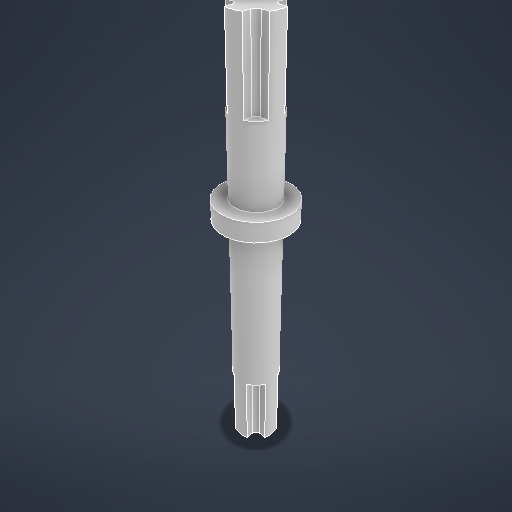
# Autodesk Inventor part: diff_gear_holder_2
Saved by Autodesk Inventor 2025 (Build 290162000, 162)
## iProperties
Created: 2024-07-25
Part Number: diff_gear_holder_2
Material: Generic
Document SubType Name: Modeling
Designer: Garfieldcmix
Density: 1 g/cm^3
Appearance: Default
Author: Garfieldcmix
Autodesk Inventor part; units mm, degrees
ref_plane "YZ Plane" through (0, 0, 0) normal (1, 0, 0) x (0, 1, 0)
ref_plane "XZ Plane" through (0, 0, 0) normal (0, 1, 0) x (-1, 0, 0)
ref_plane "XY Plane" through (0, 0, 0) normal (0, 0, 1) x (1, 0, 0)
sketch "Sketch1" plane through (0, 0, 0) normal (0, 1, 0) x (-1, 0, 0)
  line L0 (0.9, 2.4) -> (-0.9, 2.4)
  line L1 (0.9, 2.4) -> (0.9, 1.4)
  line L2 (1.4, 1.4) -> (0.9, 1.4) construction
  line L3 (1.4, 1.4) -> (1.4, 0.9) construction
  arc A0 (0.9, 1.4) -> (1.4, 0.9) centre (1.4, 1.4) ccw
  line L4 (1.4, 0.9) -> (2.4, 0.9)
  line L5 (-0.9, 1.4) -> (-0.9, 2.4)
  arc A1 (-1.4, 0.9) -> (-0.9, 1.4) centre (-1.4, 1.4) ccw
  line L6 (-2.4, 0.9) -> (-1.4, 0.9)
  line L7 (-2.4, 0.9) -> (-2.4, -0.9)
  line L8 (-1.4, -0.9) -> (-2.4, -0.9)
  arc A2 (-0.9, -1.4) -> (-1.4, -0.9) centre (-1.4, -1.4) ccw
  line L9 (-0.9, -2.4) -> (-0.9, -1.4)
  line L10 (-0.9, -2.4) -> (0.9, -2.4)
  line L11 (0.9, -1.4) -> (0.9, -2.4)
  arc A3 (1.4, -0.9) -> (0.9, -1.4) centre (1.4, -1.4) ccw
  line L12 (2.4, -0.9) -> (1.4, -0.9)
  line L13 (2.4, -0.9) -> (2.4, 0.9)
  line L14 (0, 2.4) -> (0, -2.4) construction
  circle A4 centre (0, 0) radius 2.4
  circle A5 centre (0, 0) radius 3.9
  point P0 (0, 0)
  point P1 (0, 0)
  point P2 (-2.4, 0)
  point P3 (2.4, 0)
  point P4 (2.2249, -0.9)
  point P5 (2.2249, 0.9)
  point P6 (0.9, 2.2249)
  point P7 (-0.9, 2.2249)
  point P8 (-2.2249, 0.9)
  point P9 (-2.2249, -0.9)
  point P10 (-0.9, -2.2249)
  point P11 (0.9, -2.2249)
  dimension "d6" = 1.8
  dimension "d7" = 2.4
  dimension "d8" = 1
  dimension "d9" = 0.5
  dimension "d10" = 1
  dimension "d11" = 360
  dimension "d12" = 2.4
  dimension "d13" = 0.9
  dimension "d16" = 4.8
  dimension "d24" = 7.8
  constraints: 30 end point, 8 point on circle, 6 centre point, 4 perpendicular, 3 coincident, 1 midpoint, 1 tangent, 1 vertical, 45 other
  measures "d6" distance of L0.end L1.start
  measures "d7" distance from line of point (0, 0) L0
  measures "d8" distance of L2.end L1.start
  measures "d9" distance of L2.end L3.start
  measures "d10" distance of L4.start L4.end
  measures "d12" distance from line of point (0, 0) L13
  measures "d13" distance from line of point (0, 0) L4
  measures "d16" diameter of A4
  measures "d24" diameter of A5
extrude "Extrusion2" add sketch "Sketch1" along normal blind 8 contours A4 L1 A0 L4 L12 A3 L11 L9 A2 L8 L6 A1 L5
extrude "Extrusion3" add sketch "Sketch1" along normal blind 18.1 from surface at 8 contours A4 L1 A0 L4 L12 A3 L11 L9 A2 L8 L6 A1 L5 | A4 L4 A0 L1 | L5 A1 L6 A4 | A4 L11 A3 L12 | L8 A2 L9 A4
extrude "Extrusion5" add sketch "Sketch1" along normal blind 2 from surface at 26.1 contours L1 A4 L0 | A4 L5 L0 | A4 L1 A0 L4 L12 A3 L11 L9 A2 L8 L6 A1 L5 | A4 L4 A0 L1 | L5 A1 L6 A4 | L4 L13 A4 | A4 L7 L6 | L13 L12 A4 | A4 L8 L7 | A4 L11 A3 L12 | L8 A2 L9 A4 | L11 L10 A4 | A4 L10 L9 | A5
extrude "Extrusion6" add sketch "Sketch1" along normal blind 8 from surface at 28.1 contours A4 L1 A0 L4 L12 A3 L11 L9 A2 L8 L6 A1 L5 | A4 L4 A0 L1 | L5 A1 L6 A4 | A4 L11 A3 L12 | L8 A2 L9 A4
extrude "Extrusion7" add sketch "Sketch1" along normal blind 8 from surface at 36.1 contours A4 L1 A0 L4 L12 A3 L11 L9 A2 L8 L6 A1 L5
body "Solid2"
